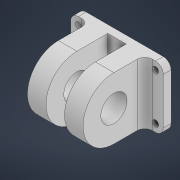
# Autodesk Inventor part: DoubleHinge
Saved by Autodesk Inventor 2021 (Build 250183000, 183)
## iProperties
Created: 2021-01-30
Part Number: DoubleHinge
Material: Generic
Document SubType Name: Modeling
Designer: PaisW
Density: 1 g/cm^3
Appearance: Default
Author: PaisW
Autodesk Inventor part; units mm, degrees
ref_plane "YZ Plane" through (0, 0, 0) normal (1, 0, 0) x (0, 1, 0)
ref_plane "XZ Plane" through (0, 0, 0) normal (0, 1, 0) x (-1, 0, 0)
ref_plane "XY Plane" through (0, 0, 0) normal (0, 0, 1) x (1, 0, 0)
sketch "Sketch8" plane through (0, 0, 0) normal (0, 0, 1) x (1, 0, 0)
  line L0 (-25, 20) -> (25, 20)
  line L1 (30, 15) -> (30, -15)
  line L2 (25, -20) -> (-25, -20)
  line L3 (-30, -15) -> (-30, 15)
  line L4 (-30, 20) -> (30, -20) construction
  line L5 (30, 20) -> (-30, -20) construction
  line L6 (-25, 15) -> (25, 15) construction
  line L7 (25, 15) -> (25, -15) construction
  line L8 (25, -15) -> (-25, -15) construction
  line L9 (-25, -15) -> (-25, 15) construction
  line L10 (-25, 15) -> (25, -15) construction
  line L11 (25, 15) -> (-25, -15) construction
  circle A0 centre (-25, 15) radius 2
  circle A1 centre (25, 15) radius 2
  circle A2 centre (25, -15) radius 2
  circle A3 centre (-25, -15) radius 2
  arc A4 (-25, 20) -> (-30, 15) centre (-25, 15) ccw
  arc A5 (-30, -15) -> (-25, -20) centre (-25, -15) ccw
  arc A6 (25, -20) -> (30, -15) centre (25, -15) ccw
  arc A7 (30, 15) -> (25, 20) centre (25, 15) ccw
  point P0 (0, 0)
  dimension "d30" = 40
  dimension "d31" = 4
  dimension "d32" = 50
  dimension "d33" = 60
  dimension "d34" = 30
  dimension "d35" = 5
  constraints: 24 end point, 8 centre point, 8 point on circle, 8 point on line, 8 tangent, 6 equal radius, 4 coincident, 4 midpoint, 4 parallel, 2 horizontal, 2 perpendicular
  measures "d30" distance of L5.start L4.end
  measures "d31" diameter of A0
  measures "d32" distance of L7.end L8.end
  measures "d33" distance of L4.end L5.end
  measures "d34" distance of L6.end L7.end
  measures "d35" radius of A4
extrude "Extrusion8" add sketch "Sketch8" along normal blind 5
sketch "Sketch9" plane through (0, 0, 5) normal (0, 0, 1) x (1, 0, 0)
  line L0 (-25, -20) -> (25, -20) projected
  line L1 (-18, 20) -> (-6, 20)
  line L2 (-6, 20) -> (-6, -20)
  line L3 (-6, -20) -> (-18, -20)
  line L4 (-18, -20) -> (-18, 20)
  line L5 (-18, 20) -> (-6, -20) construction
  line L6 (-6, 20) -> (-18, -20) construction
  line L7 (6, 20) -> (18, 20)
  line L8 (18, 20) -> (18, -20)
  line L9 (18, -20) -> (6, -20)
  line L10 (6, -20) -> (6, 20)
  line L11 (6, 20) -> (18, -20) construction
  line L12 (18, 20) -> (6, -20) construction
  line L13 (25, 20) -> (-25, 20) projected
  point P0 (0, 0)
  point P1 (-12, 0)
  point P2 (12, 0)
  dimension "d38" = 12
  dimension "d39" = 6
  dimension "d40" = 6
  constraints: 24 end point, 4 midpoint, 4 parallel, 3 collinear, 2 horizontal, 2 perpendicular, 2 point on line
  measures "d38" distance of L1.start L1.end
  measures "d39" distance from line of point (0, 0) L2
  measures "d40" distance from line of point (0, 0) L10
extrude "Extrusion9" add sketch "Sketch9" along normal blind 40 contours L4 L1 L2 L0 | L10 L7 L8 L0
fillet "Fillet3" radius 5 2 edges at (-18, 0, 5) (18, 0, 5)
sketch "Sketch10" plane through (18, -20, 45) normal (1, 0, 0) x (0, 0, -1)
  circle A0 centre (20, 20) radius 8.5
  circle A1 centre (20, 20) radius 20
  line L0 (0, 0) -> (0, 40)
  line L1 (38.3283, 0) -> (41.7977, 39.6968)
  line L2 (20, 0) -> (0, 0)
  line L3 (20, 0) -> (0, 0)
  line L4 (0, 0) -> (0, 40)
  line L5 (0, 40) -> (20, 40)
  line L6 (35, 40) -> (0, 40) projected
  line L7 (0, 0) -> (0, 40) projected
  line L8 (35, 0) -> (0, 0) projected
  point P0 (45, 20)
  point P1 (45, 20)
  point P2 (0, 20)
  dimension "d44" = 17
  constraints: 13 end point, 6 tangent, 2 centre point, 2 perpendicular, 2 point on circle, 1 coincident, 1 collinear
  measures "d44" diameter of A0
extrude "Extrusion10" cut sketch "Sketch10" against normal through all contours A0 | A1 L0 L5 | A1 L2 L0
sketch "Sketch5" plane through (0, 0, 0) normal (0, 0, 1) x (1, 0, 0)
  line L0 (15, 15) -> (15, -15) construction
  line L1 (15, -15) -> (-15, -15) construction
  line L2 (-15, -15) -> (-15, 15) construction
  line L3 (-15, 15) -> (15, -15) construction
  line L4 (15, 15) -> (-15, -15) construction
  circle A0 centre (-15, 15) radius 2
  circle A1 centre (15, 15) radius 2
  circle A2 centre (15, -15) radius 2
  circle A3 centre (-15, -15) radius 2
  line L5 (-15, 20) -> (15, 20)
  line L6 (20, 15) -> (20, -15)
  line L7 (15, -20) -> (-15, -20)
  line L8 (-20, -15) -> (-20, 15)
  line L9 (-20, 20) -> (20, -20) construction
  line L10 (20, 20) -> (-20, -20) construction
  arc A4 (20, 15) -> (15, 20) centre (15, 15) ccw
  arc A5 (15, -20) -> (20, -15) centre (15, -15) ccw
  arc A6 (-20, -15) -> (-15, -20) centre (-15, -15) ccw
  arc A7 (-15, 20) -> (-20, 15) centre (-15, 15) ccw
  point P0 (0, 0)
  dimension "d16" = 4
  dimension "d17" = 30
  dimension "d18" = 40
  dimension "d20" = 5
  constraints: 22 end point, 9 point on line, 8 centre point, 8 point on circle, 8 tangent, 6 equal radius, 4 coincident, 4 midpoint, 3 parallel, 2 perpendicular, 1 horizontal
  measures "d16" diameter of A0
  measures "d17" distance of L1.end L2.end
  measures "d18" distance of L9.end L10.end
  measures "d20" radius of A4
sketch "Sketch6" plane through (0, 0, 10) normal (0, 0, 1) x (1, 0, 0)
  line L0 (-15, -20) -> (15, -20) projected
  line L1 (-6, 20) -> (6, 20)
  line L2 (6, 20) -> (6, -20)
  line L3 (6, -20) -> (-6, -20)
  line L4 (-6, -20) -> (-6, 20)
  line L5 (-6, 20) -> (6, -20) construction
  line L6 (6, 20) -> (-6, -20) construction
  point P0 (0, 0)
  dimension "d23" = 12
  constraints: 12 end point, 2 midpoint, 2 parallel, 1 horizontal, 1 perpendicular, 1 point on line
  measures "d23" distance of L1.start L1.end
sketch "Sketch7" plane through (6, -20, 50) normal (1, 0, 0) x (0, 0, -1)
  circle A0 centre (20, 20) radius 8.5
  circle A1 centre (20, 20) radius 20
  line L0 (0, 0) -> (0, 40) projected
  line L1 (40, 0) -> (40, 40) projected
  line L2 (35, 0) -> (0, 0) projected
  line L3 (20, 0) -> (0, 0)
  line L4 (0, 0) -> (0, 40)
  line L5 (0, 40) -> (20, 40)
  line L6 (35, 40) -> (0, 40) projected
  point P0 (50, 20)
  point P1 (0, 20)
  dimension "d27" = 17
  constraints: 6 end point, 3 tangent, 2 centre point, 2 point on circle, 2 point on line, 1 coincident, 1 collinear
  measures "d27" diameter of A0
sketch "Sketch1" plane through (0, 0, 0) normal (0, 1, 0) x (-1, 0, 0)
  line L0 (27.5, 22.5) -> (-27.5, 22.5)
  line L1 (-27.5, 22.5) -> (-27.5, -22.5)
  line L2 (-27.5, -22.5) -> (27.5, -22.5)
  line L3 (27.5, -22.5) -> (27.5, 22.5)
  point P0 (0, 0)
  point P1 (27.5, 0)
  point P2 (0, -22.5)
  dimension "d0" = 45
  dimension "d1" = 55
  constraints: 8 end point, 2 midpoint, 2 parallel, 1 horizontal, 1 horizontal alignment, 1 perpendicular, 1 vertical alignment
  measures "d0" distance of L2.end L0.start
  measures "d1" distance of L1.end L2.end
sketch "Sketch2" plane through (0, 10, 0) normal (0, 1, 0) x (1, 0, 0)
  line L0 (-27.5, 22.5) -> (-27.5, -22.5) projected
  line L1 (-27.5, -22.5) -> (27.5, -22.5) projected
  line L2 (-27.5, 22.5) -> (-19.5, 22.5)
  line L3 (-19.5, 22.5) -> (-19.5, -22.5)
  line L4 (-19.5, -22.5) -> (-27.5, -22.5)
  line L5 (-27.5, -22.5) -> (-27.5, 22.5)
  line L6 (27.5, -22.5) -> (27.5, 22.5) projected
  line L7 (27.5, 22.5) -> (19.5, 22.5)
  line L8 (19.5, 22.5) -> (19.5, -22.5)
  line L9 (19.5, -22.5) -> (27.5, -22.5)
  line L10 (27.5, -22.5) -> (27.5, 22.5)
  point P0 (0, 0)
  dimension "d4" = 8
  dimension "d5" = 8
  constraints: 16 end point, 4 parallel, 2 horizontal, 2 perpendicular, 2 point on line
  measures "d4" distance between parallel lines of L0 L3
  measures "d5" distance between parallel lines of L6 L8
sketch "Sketch4" plane through (0, 0, 0) normal (0, -1, 0) x (1, 0, 0)
  line L0 (15, 15) -> (-15, 15) construction
  line L1 (-15, 15) -> (-15, -15) construction
  line L2 (-15, -15) -> (15, -15) construction
  line L3 (15, -15) -> (15, 15) construction
  line L4 (15, 15) -> (-15, -15) construction
  line L5 (-15, 15) -> (15, -15) construction
  circle A0 centre (15, -15) radius 2
  circle A1 centre (-15, -15) radius 2
  circle A2 centre (-15, 15) radius 2
  circle A3 centre (15, 15) radius 2
  point P0 (0, 0)
  dimension "d12" = 30
  dimension "d13" = 4
  constraints: 12 end point, 4 centre point, 4 coincident, 3 equal radius, 2 midpoint, 2 parallel, 2 perpendicular, 1 horizontal
  measures "d12" distance of L0.end L1.end
  measures "d13" diameter of A0
sketch "Sketch3" plane through (27.5, 0, 22.5) normal (1, 0, 0) x (0, 0, -1)
  circle A0 centre (22.5, 25) radius 15
  line L0 (22.5, 25) -> (22.5, 47.5) construction
  line L1 (45, 47.5) -> (0, 47.5) projected
  line L2 (22.5, 25) -> (45, 25) construction
  line L3 (45, 0) -> (45, 47.5) projected
  point P0 (22.5, 0)
  dimension "d9" = 30
  constraints: 4 end point, 1 centre point, 1 horizontal, 1 midpoint, 1 perpendicular, 1 point on line, 1 vertical alignment
  measures "d9" diameter of A0
body "Solid1"
body "Solid2"
body "Solid3"
